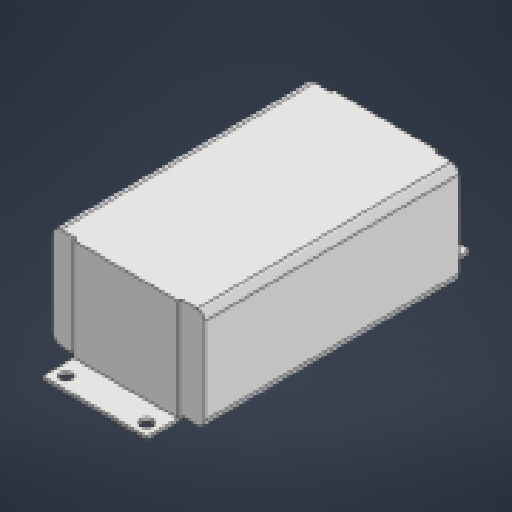
# Autodesk Inventor part: esc
Saved by Autodesk Inventor 2024 (Build 280153000, 153)
## iProperties
Created: 2024-05-03
Part Number: esc
Material: Generic
Document SubType Name: Modeling
Designer: markm
Density: 1 g/cm^3
Appearance: Default
Author: markm
Autodesk Inventor part; units mm, degrees
ref_plane "YZ Plane" through (0, 0, 0) normal (1, 0, 0) x (0, 1, 0)
ref_plane "XZ Plane" through (0, 0, 0) normal (0, 1, 0) x (-1, 0, 0)
ref_plane "XY Plane" through (0, 0, 0) normal (0, 0, 1) x (1, 0, 0)
sketch "Sketch1" plane through (0, 0, 0) normal (0, 0, 1) x (1, 0, 0)
  line L0 (-25.35, -16.9) -> (25.35, -16.9)
  line L1 (25.35, -16.9) -> (25.35, 16.9)
  line L2 (25.35, 16.9) -> (-25.35, 16.9)
  line L3 (-25.35, 16.9) -> (-25.35, -16.9)
  line L4 (-25.35, -16.9) -> (25.35, 16.9) construction
  line L5 (25.35, -16.9) -> (-25.35, 16.9) construction
  point P0 (0, 0)
  dimension "d0" = 50.7
  dimension "d1" = 33.8
  constraints: 12 end point, 2 midpoint, 2 parallel, 1 horizontal, 1 perpendicular
  measures "d0" distance of L2.end L1.end
  measures "d1" distance of L1.end L0.end
extrude "Extrusion1" add sketch "Sketch1" along normal blind 42.5
sketch "Sketch3" plane through (0, 0, 0) normal (1, 0, 0) x (0, 1, 0)
  line L0 (16.9, 42.5) -> (16.9, 0) projected
  line L1 (16.9, 0) -> (-16.9, 0) projected
  line L2 (-16.9, 0) -> (-16.9, 42.5) projected
  line L3 (-16.9, 42.5) -> (16.9, 42.5) projected
  line L4 (16.9, 42.5) -> (16.9, 43.5)
  line L5 (16.9, 43.5) -> (-17.1, 43.5)
  line L6 (-17.1, 43.5) -> (-17.1, 54)
  line L7 (-17.1, 54) -> (-18.1, 54)
  line L8 (-18.1, 54) -> (-18.1, 43.5)
  line L9 (-17.1, 42.5) -> (-16.9, 42.5)
  arc A0 (-18.1, 43.5) -> (-17.1, 42.5) centre (-17.1, 43.5) ccw
  point P0 (0, 0)
  dimension "d4" = 1
  dimension "d5" = 1
  dimension "d6" = 35
  dimension "d7" = 1
  dimension "d8" = 54
  constraints: 12 end point, 5 perpendicular, 2 point on circle, 2 tangent, 1 centre point, 1 vertical
  measures "d4" distance between parallel lines of L3 L5
  measures "d5" distance between parallel lines of L8 L6
  measures "d6" distance between parallel lines of L4 L8
  measures "d7" radius of A0
  measures "d8" distance between parallel lines of L1 L7
extrude "Extrusion2" add sketch "Sketch3" along normal mid plane 35 contours L3 L9 A0 L8 L7 L6 L5 L4
fillet "Fillet2" radius 2.5 4 edges at (25.35, -16.9, 21.25) (25.35, 16.9, 21.25) (-25.35, 16.9, 21.25) (-25.35, -16.9, 21.25)
sketch "Sketch4" plane through (-17.5, -17.1, 54) normal (0, 1, 0) x (1, 0, 0)
  line L0 (17.5, 54) -> (17.5, 4) construction
  line L1 (4, 4) -> (31, 4) construction
  circle A0 centre (4, 4) radius 2
  circle A1 centre (31, 4) radius 2
  dimension "d13" = 4
  dimension "d14" = 50
  dimension "d15" = 27
  constraints: 4 end point, 3 coincident, 2 centre point, 1 equal radius, 1 horizontal, 1 midpoint, 1 vertical
  measures "d13" diameter of A0
  measures "d14" distance of L0.start L0.end
  measures "d15" distance of L1.end L1.start
extrude "Extrusion3" cut sketch "Sketch4" against normal through all
mirror "Mirror1" about plane through (0, 0, 0) normal (0, 0, 1)
body "Solid1"
